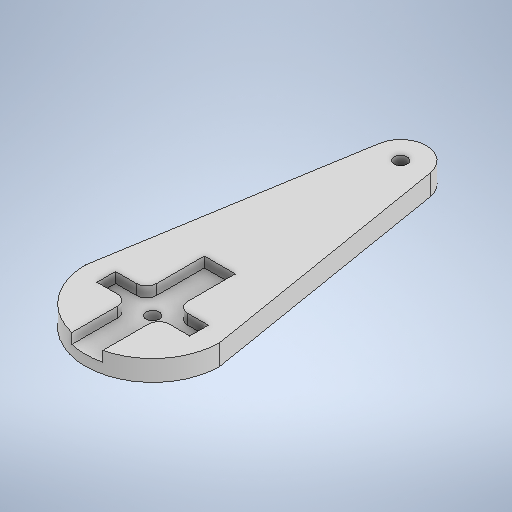
# Autodesk Inventor part: 6P-016
Saved by Autodesk Inventor 2025.2 (Build 292293000, 293)
## iProperties
Created: 2025-01-15
Part Number: 6P-016
Material: Generic
Document SubType Name: Modeling
Designer: Sameer Alhindi
Density: 1 g/cm^3
Appearance: Default
Author: Sameer Alhindi
Autodesk Inventor part; units mm, degrees
ref_plane "YZ Plane" through (0, 0, 0) normal (1, 0, 0) x (0, 1, 0)
ref_plane "XZ Plane" through (0, 0, 0) normal (0, 1, 0) x (-1, 0, 0)
ref_plane "XY Plane" through (0, 0, 0) normal (0, 0, 1) x (1, 0, 0)
sketch "Sketch1" plane through (0, 0, 0) normal (0, 1, 0) x (-1, 0, 0)
  arc A0 (13, 0) -> (-13, 0) centre (0, 0) ccw
  circle A1 centre (0, 0) radius 1.25
  arc A2 (-4.9331, -48.8152) -> (4.9331, -48.8152) centre (0, -48) ccw
  line L0 (13, 0) -> (4.9331, -48.8152)
  line L1 (-13, 0) -> (-4.9331, -48.8152)
  circle A3 centre (0, -48) radius 1.25
  dimension "d3" = 2.5
  dimension "d16" = 10
  dimension "d17" = 2.5
  dimension "d19" = 13
  dimension "d20" = 48
  constraints: 4 centre point, 4 end point, 4 point on circle, 3 coincident, 2 tangent, 1 vertical alignment
  measures "d3" diameter of A1
  measures "d16" diameter of A2
  measures "d17" diameter of A3
  measures "d19" radius of A0
  measures "d20" distance of A2.centre point (0, 0)
extrude "Extrusion1" add sketch "Sketch1" along normal blind 4
sketch "Sketch2" plane through (0, 4, 0) normal (0, 1, 0) x (1, 0, 0)
  line L0 (-3, -13) -> (3, -13)
  line L1 (3, 13) -> (-3, 13)
  circle A0 centre (0, 0) radius 1.25 projected
  line L2 (-3, -13) -> (3, 13) construction
  line L3 (3, -13) -> (-3, 13) construction
  line L4 (9, 1.7894) -> (9, -1.8106)
  line L5 (-9, -1.7894) -> (-9, 1.8106)
  line L6 (-9, 1.8106) -> (9, -1.8106) construction
  line L7 (9, 1.7894) -> (-9, -1.7894) construction
  line L8 (3, 1.7894) -> (9, 1.7894)
  line L9 (-9, 1.8106) -> (-3, 1.8106)
  line L10 (-3, -1.7894) -> (-9, -1.7894)
  line L11 (9, -1.8106) -> (3, -1.8106)
  line L12 (3, 1.7894) -> (3, 13)
  line L13 (3, -13) -> (3, -1.8106)
  line L14 (-3, -1.7894) -> (-3, -13)
  line L15 (-3, 13) -> (-3, 1.8106)
  point P0 (-9, 0.0106)
  dimension "d7" = 6
  dimension "d12" = 3.6
  dimension "d13" = 13
  dimension "d14" = 13
  dimension "d15" = 9
  constraints: 32 end point, 10 parallel, 5 midpoint, 4 perpendicular, 3 horizontal
  measures "d7" distance of L1.end L1.start
  measures "d12" distance between parallel lines of L10 L9
  measures "d13" distance from line of L1 point (0, 0)
  measures "d14" distance from line of L0 point (0, 0)
  measures "d15" distance of point (0, 0) point (-9, 0.011)
extrude "Extrusion2" cut sketch "Sketch2" against normal blind 2 contours L14 L10 L5 L9 L15 L1 L12 L8 L4 L11 L13 L0 | A0
fillet "Fillet3" radius 2 4 edges at (-3, 3, -1.8106) (-3, 3, 1.7894) (3, 3, -1.7894) (3, 3, 1.8106)
body "Solid1"
